Autodesk Fusion 360 part; units mm, degrees
(part 2 of 2)
sketch "Sketch15" plane through (0, 0, 3) normal (0, 0, 1) x (-1, 0, 0)
  line L0 (-1.3462, 92.3209) -> (-1.3462, 60.3952)
  line L1 (-1.3462, 60.3952) -> (-51.7, 11.7691)
  line L2 (-51.7, 11.7691) -> (-51.7, -47.6791)
  line L3 (-51.7, -47.6791) -> (-52.7, -47.6791)
  line L4 (-52.7, -47.6791) -> (-52.7, 12.1936)
  line L5 (-52.7, 12.1936) -> (-2.3462, 60.8196)
  line L6 (-2.3462, 60.8196) -> (-2.3462, 92.3209)
  line L7 (-2.3462, 92.3209) -> (-4.4462, 92.3209)
  line L8 (-4.4462, 92.3209) -> (-4.4462, 61.711)
  line L9 (-4.4462, 61.711) -> (-54.8, 13.085)
  line L10 (-54.8, 13.085) -> (-54.8, -47.6791)
  line L11 (-54.8, -47.6791) -> (-55.8, -47.6791)
  line L12 (-55.8, -47.6791) -> (-55.8, -26.7291)
  line L13 (-55.8, -26.7291) -> (-58.8, -26.7291)
  line L14 (-58.8, -26.7291) -> (-58.8, -18.6291)
  line L15 (-58.8, -18.6291) -> (-55.8, -18.6291)
  line L16 (-55.8, -18.6291) -> (-55.8, 13.5094)
  line L17 (-55.8, 13.5094) -> (-33.2311, 35.304)
  line L18 (-33.2311, 35.304) -> (-35.3151, 37.462)
  line L19 (-35.3151, 37.462) -> (-29.4884, 43.0887)
  line L20 (-29.4884, 43.0887) -> (-27.4044, 40.9307)
  line L21 (-27.4044, 40.9307) -> (-5.4462, 62.1355)
  line L22 (-5.4462, 62.1355) -> (-5.4462, 77.7709)
  line L23 (-5.4462, 77.7709) -> (-8.4462, 77.7709)
  line L24 (-8.4462, 77.7709) -> (-8.4462, 85.8709)
  line L25 (-8.4462, 85.8709) -> (-5.4462, 85.8709)
  line L26 (-5.4462, 85.8709) -> (-5.4462, 92.3209)
  line L27 (-5.4462, 92.3209) -> (-12.45, 92.3209)
  line L28 (-12.45, 92.3209) -> (-12.45, 88.3209)
  line L29 (-12.45, 88.3209) -> (-20.55, 88.3209)
  line L30 (-20.55, 88.3209) -> (-20.55, 92.3209)
  line L31 (-20.55, 92.3209) -> (-71.45, 92.3209)
  line L32 (-71.45, 92.3209) -> (-71.45, 88.3209)
  line L33 (-71.45, 88.3209) -> (-79.55, 88.3209)
  line L34 (-79.55, 88.3209) -> (-79.55, 92.3209)
  line L35 (-79.55, 92.3209) -> (-86.5, 92.3209)
  line L36 (-86.5, 92.3209) -> (-86.5, 85.8709)
  line L37 (-86.5, 85.8709) -> (-82.5, 85.8709)
  line L38 (-82.5, 85.8709) -> (-82.5, 77.7709)
  line L39 (-82.5, 77.7709) -> (-86.5, 77.7709)
  line L40 (-86.5, 77.7709) -> (-86.5, 5.6048)
  line L41 (-86.5, 5.6048) -> (-82.5, 5.6048)
  line L42 (-82.5, 5.6048) -> (-82.5, -2.4952)
  line L43 (-82.5, -2.4952) -> (-86.5, -2.4952)
  line L44 (-86.5, -2.4952) -> (-86.5, -73.6699)
  line L45 (-86.5, -73.6699) -> (-82.5, -73.6699)
  line L46 (-82.5, -73.6699) -> (-82.5, -81.7699)
  line L47 (-82.5, -81.7699) -> (-86.5, -81.7699)
  line L48 (-86.5, -81.7699) -> (-86.5, -88.2199)
  line L49 (-86.5, -88.2199) -> (-79.55, -88.2199)
  line L50 (-79.55, -88.2199) -> (-79.55, -84.2199)
  line L51 (-79.55, -84.2199) -> (-71.45, -84.2199)
  line L52 (-71.45, -84.2199) -> (-71.45, -88.2199)
  line L53 (-71.45, -88.2199) -> (-51.55, -88.2199)
  line L54 (-51.55, -88.2199) -> (-51.55, -84.2199)
  line L55 (-51.55, -84.2199) -> (-43.45, -84.2199)
  line L56 (-43.45, -84.2199) -> (-43.45, -88.2199)
  line L57 (-43.45, -88.2199) -> (-36.5, -88.2199)
  line L58 (-36.5, -88.2199) -> (-36.5, -87.7699)
  line L59 (-36.5, -87.7699) -> (-40.5, -87.7699)
  line L60 (-40.5, -87.7699) -> (-40.5, -79.6699)
  line L61 (-40.5, -79.6699) -> (-36.5, -79.6699)
  line L62 (-36.5, -79.6699) -> (-36.5, -71.6718)
  line L63 (-36.5, -71.6718) -> (-40.5, -71.6718)
  line L64 (-40.5, -71.6718) -> (-40.5, -63.5718)
  line L65 (-40.5, -63.5718) -> (-36.5, -63.5718)
  line L66 (-36.5, -63.5718) -> (-36.5, -63.2199)
  line L67 (-36.5, -63.2199) -> (-36.2957, -62.8659)
  line L68 (-36.2957, -62.8659) -> (-39.7598, -60.8659)
  line L69 (-39.7598, -60.8659) -> (-35.7098, -53.8511)
  line L70 (-35.7098, -53.8511) -> (-32.2457, -55.8511)
  line L71 (-32.2457, -55.8511) -> (-4.298, -7.4443)
  line L72 (-4.298, -7.4443) -> (-7.7621, -5.4443)
  line L73 (-7.7621, -5.4443) -> (-3.7121, 1.5705)
  line L74 (-3.7121, 1.5705) -> (-0.248, -0.4295)
  line L75 (-0.248, -0.4295) -> (0, 0)
  line L76 (0, 0) -> (0.466, 0.1696)
  line L77 (0.466, 0.1696) -> (-0.902, 3.9284)
  line L78 (-0.902, 3.9284) -> (6.7095, 6.6988)
  line L79 (6.7095, 6.6988) -> (8.0776, 2.94)
  line L80 (8.0776, 2.94) -> (80.344, 29.2428)
  line L81 (80.344, 29.2428) -> (78.9759, 33.0016)
  line L82 (78.9759, 33.0016) -> (86.5874, 35.772)
  line L83 (86.5874, 35.772) -> (87.9555, 32.0132)
  line L84 (87.9555, 32.0132) -> (88.801, 32.3209)
  line L85 (88.801, 32.3209) -> (88.801, 36.2709)
  line L86 (88.801, 36.2709) -> (84.801, 36.2709)
  line L87 (84.801, 36.2709) -> (84.801, 44.3709)
  line L88 (84.801, 44.3709) -> (88.801, 44.3709)
  line L89 (88.801, 44.3709) -> (88.801, 83.7709)
  line L90 (88.801, 83.7709) -> (84.801, 83.7709)
  line L91 (84.801, 83.7709) -> (84.801, 91.8709)
  line L92 (84.801, 91.8709) -> (88.801, 91.8709)
  line L93 (88.801, 91.8709) -> (88.801, 92.3209)
  line L94 (88.801, 92.3209) -> (81.851, 92.3209)
  line L95 (81.851, 92.3209) -> (81.851, 88.3209)
  line L96 (81.851, 88.3209) -> (73.751, 88.3209)
  line L97 (73.751, 88.3209) -> (73.751, 92.3209)
  line L98 (73.751, 92.3209) -> (-1.3462, 92.3209)
  line L99 (75, 65) -> (70, 65)
  line L100 (70, 65) -> (70, 40)
  line L101 (70, 40) -> (75, 40)
  line L102 (75, 40) -> (75, 65)
  line L103 (75, 40) -> (35, 40)
  line L104 (35, 40) -> (35, 45)
  line L105 (35, 45) -> (75, 45)
  line L106 (75, 45) -> (75, 40)
  line L107 (65, 50) -> (60, 50)
  line L108 (60, 50) -> (60, 65)
  line L109 (60, 65) -> (65, 65)
  line L110 (65, 65) -> (65, 50)
  line L111 (55, 45) -> (50, 45)
  line L112 (50, 45) -> (50, 55)
  line L113 (50, 55) -> (55, 55)
  line L114 (55, 55) -> (55, 45)
  line L115 (55, 55) -> (35, 55)
  line L116 (35, 55) -> (35, 50)
  line L117 (35, 50) -> (55, 50)
  line L118 (55, 50) -> (55, 55)
  line L119 (35, 50) -> (40, 50)
  line L120 (40, 50) -> (40, 65)
  line L121 (40, 65) -> (35, 65)
  line L122 (35, 65) -> (35, 50)
  line L123 (35, 65) -> (65, 65)
  line L124 (65, 65) -> (65, 60)
  line L125 (65, 60) -> (35, 60)
  line L126 (35, 60) -> (35, 65)
  line L127 (30, 40) -> (25, 40)
  line L128 (25, 40) -> (25, 45)
  line L129 (25, 45) -> (30, 45)
  line L130 (30, 45) -> (30, 40)
  line L131 (30, 50) -> (25, 50)
  line L132 (25, 50) -> (25, 55)
  line L133 (25, 55) -> (30, 55)
  line L134 (30, 55) -> (30, 50)
  line L135 (30, 60) -> (25, 60)
  line L136 (25, 60) -> (25, 65)
  line L137 (25, 65) -> (30, 65)
  line L138 (30, 65) -> (30, 60)
  line L139 (74.99, 67.4454) -> (74.0541, 67.4454)
  line L140 (74.0541, 67.4454) -> (72.8031, 71.0457)
  line L141 (72.8031, 71.0457) -> (72.784, 71.0457)
  line L142 (72.784, 71.0457) -> (71.5425, 67.4454)
  line L143 (71.5425, 67.4454) -> (70.597, 67.4454)
  line L144 (70.597, 67.4454) -> (70.597, 74.245)
  line L145 (70.597, 74.245) -> (71.5711, 74.245)
  line L146 (71.5711, 74.245) -> (71.5711, 70.1098)
  line L147 (71.5711, 70.1098) -> (71.5902, 70.1098)
  line L148 (71.5902, 70.1098) -> (72.5548, 73.0321)
  line L149 (72.5548, 73.0321) -> (73.0418, 73.0321)
  line L150 (73.0418, 73.0321) -> (73.9968, 70.1098)
  line L151 (73.9968, 70.1098) -> (74.0159, 70.1098)
  line L152 (74.0159, 70.1098) -> (74.0159, 74.245)
  line L153 (74.0159, 74.245) -> (74.99, 74.245)
  line L154 (74.99, 74.245) -> (74.99, 67.4454)
  line L155 (69.6515, 67.4454) -> (68.6775, 67.4454)
  line L156 (68.6775, 67.4454) -> (68.6775, 74.245)
  line L157 (68.6775, 74.245) -> (69.6515, 74.245)
  line L158 (69.6515, 74.245) -> (69.6515, 67.4454)
  line L159 (67.732, 67.4454) -> (66.7579, 67.4454)
  line L160 (66.7579, 67.4454) -> (66.7579, 73.2709)
  line L161 (66.7579, 73.2709) -> (64.8288, 73.2709)
  line L162 (64.8288, 73.2709) -> (64.8288, 74.245)
  line L163 (64.8288, 74.245) -> (67.732, 74.245)
  line L164 (67.732, 74.245) -> (67.732, 67.4454)
  line L165 (64.1985, 67.4454) -> (61.2953, 67.4454)
  line L166 (61.2953, 67.4454) -> (61.2953, 68.3622)
  line L167 (61.2953, 68.3622) -> (63.2244, 68.3622)
  line L168 (63.2244, 68.3622) -> (63.2244, 70.3581)
  line L169 (63.2244, 70.3581) -> (61.5436, 70.3581)
  line L170 (61.5436, 70.3581) -> (61.5436, 71.2749)
  line L171 (61.5436, 71.2749) -> (63.2244, 71.2749)
  line L172 (63.2244, 71.2749) -> (63.2244, 73.2709)
  line L173 (63.2244, 73.2709) -> (61.2953, 73.2709)
  line L174 (61.2953, 73.2709) -> (61.2953, 74.245)
  line L175 (61.2953, 74.245) -> (64.1985, 74.245)
  line L176 (64.1985, 74.245) -> (64.1985, 67.4454)
  line L177 (57.5135, 69.4031) -> (58.4876, 69.4031)
  line L178 (58.4876, 69.4031) -> (58.4876, 69.1835)
  spline S0 degree 3 poles (58.4876, 69.1835) (58.4932, 69.0777) (58.5041, 68.8742) (58.6026, 68.6961) (58.65, 68.6105) knots 0 0 0 0 0.031302 0.06025 0.06025 0.06025 0.06025
  spline S1 degree 3 poles (58.65, 68.6105) (58.7141, 68.5382) (58.8526, 68.382) (59.0625, 68.3691) (59.1752, 68.3622) knots 0 0 0 0 0.027897 0.060252 0.060252 0.060252 0.060252
  spline S2 degree 3 poles (59.1752, 68.3622) (59.2375, 68.3644) (59.354, 68.3685) (59.4601, 68.4163) (59.5095, 68.4386) knots 0 0 0 0 0.018483 0.034579 0.034579 0.034579 0.034579
  spline S3 degree 3 poles (59.5095, 68.4386) (59.5488, 68.466) (59.6276, 68.5209) (59.6825, 68.5997) (59.71, 68.6391) knots 0 0 0 0 0.014281 0.028562 0.028562 0.028562 0.028562
  spline S4 degree 3 poles (59.71, 68.6391) (59.7309, 68.6807) (59.7752, 68.7686) (59.795, 68.8651) (59.8055, 68.9161) knots 0 0 0 0 0.013891 0.029409 0.029409 0.029409 0.029409
  spline S5 degree 3 poles (59.8055, 68.9161) (59.8139, 68.9685) (59.831, 69.076) (59.8331, 69.1849) (59.8342, 69.2408) knots 0 0 0 0 0.015903 0.032631 0.032631 0.032631 0.032631
  spline S6 degree 3 poles (59.8342, 69.2408) (59.8339, 69.3029) (59.8334, 69.4175) (59.8274, 69.5321) (59.8246, 69.5846) knots 0 0 0 0 0.018624 0.034398 0.034398 0.034398 0.034398
  spline S7 degree 3 poles (59.8246, 69.5846) (59.817, 69.6274) (59.8021, 69.7104) (59.7658, 69.7865) (59.7482, 69.8233) knots 0 0 0 0 0.012974 0.025169 0.025169 0.025169 0.025169
  spline S8 degree 3 poles (59.7482, 69.8233) (59.7265, 69.8548) (59.6812, 69.9204) (59.6185, 69.9696) (59.5858, 69.9952) knots 0 0 0 0 0.011413 0.023766 0.023766 0.023766 0.023766
  spline S9 degree 3 poles (59.5858, 69.9952) (59.5418, 70.0217) (59.444, 70.0806) (59.3383, 70.1241) (59.2803, 70.148) knots 0 0 0 0 0.015399 0.03421 0.03421 0.03421 0.03421
  line L179 (59.2803, 70.148) -> (58.5353, 70.4441)
  spline S10 degree 3 poles (58.5353, 70.4441) (58.435, 70.4852) (58.2475, 70.562) (58.0855, 70.6836) (58.0101, 70.7401) knots 0 0 0 0 0.032366 0.060512 0.060512 0.060512 0.060512
  spline S11 degree 3 poles (58.0101, 70.7401) (57.9473, 70.7968) (57.8226, 70.9095) (57.7437, 71.0579) (57.7045, 71.1317) knots 0 0 0 0 0.025155 0.050009 0.050009 0.050009 0.050009
  spline S12 degree 3 poles (57.7045, 71.1317) (57.6692, 71.2102) (57.5951, 71.3752) (57.5666, 71.5538) (57.5517, 71.6474) knots 0 0 0 0 0.025714 0.053996 0.053996 0.053996 0.053996
  spline S13 degree 3 poles (57.5517, 71.6474) (57.5406, 71.7499) (57.5168, 71.9689) (57.5146, 72.1892) (57.5135, 72.3063) knots 0 0 0 0 0.030932 0.066041 0.066041 0.066041 0.066041
  spline S14 degree 3 poles (57.5135, 72.3063) (57.5166, 72.4452) (57.5227, 72.7151) (57.5744, 72.98) (57.5994, 73.1085) knots 0 0 0 0 0.041598 0.080809 0.080809 0.080809 0.080809
  spline S15 degree 3 poles (57.5994, 73.1085) (57.6319, 73.2242) (57.695, 73.4491) (57.8235, 73.6441) (57.8859, 73.7388) knots 0 0 0 0 0.035787 0.069609 0.069609 0.069609 0.069609
  spline S16 degree 3 poles (57.8859, 73.7388) (57.9567, 73.8211) (58.1024, 73.9906) (58.3, 74.0955) (58.4017, 74.1495) knots 0 0 0 0 0.032249 0.06644 0.06644 0.06644 0.06644
  spline S17 degree 3 poles (58.4017, 74.1495) (58.5206, 74.194) (58.7758, 74.2895) (59.0486, 74.2978) (59.1943, 74.3023) knots 0 0 0 0 0.037829 0.081211 0.081211 0.081211 0.081211
  spline S18 degree 3 poles (59.1943, 74.3023) (59.3092, 74.2975) (59.5349, 74.2881) (59.7484, 74.2143) (59.8532, 74.1781) knots 0 0 0 0 0.034282 0.067373 0.067373 0.067373 0.067373
  spline S19 degree 3 poles (59.8532, 74.1781) (59.9507, 74.1339) (60.1417, 74.0473) (60.3007, 73.9107) (60.3785, 73.8439) knots 0 0 0 0 0.031927 0.06254 0.06254 0.06254 0.06254
  spline S20 degree 3 poles (60.3785, 73.8439) (60.4484, 73.7669) (60.5898, 73.6112) (60.6841, 73.4232) (60.7318, 73.3282) knots 0 0 0 0 0.031027 0.062774 0.062774 0.062774 0.062774
  spline S21 degree 3 poles (60.7318, 73.3282) (60.7681, 73.2265) (60.8418, 73.0196) (60.8512, 72.8) (60.856, 72.6883) knots 0 0 0 0 0.032175 0.065507 0.065507 0.065507 0.065507
  line L180 (60.856, 72.6883) -> (60.856, 72.3254)
  line L181 (60.856, 72.3254) -> (59.8819, 72.3254)
  line L182 (59.8819, 72.3254) -> (59.8819, 72.631)
  spline S22 degree 3 poles (59.8819, 72.631) (59.8755, 72.7182) (59.8628, 72.8925) (59.7737, 73.0429) (59.7291, 73.1181) knots 0 0 0 0 0.02583 0.051669 0.051669 0.051669 0.051669
  spline S23 degree 3 poles (59.7291, 73.1181) (59.6611, 73.1792) (59.5103, 73.3147) (59.3063, 73.3234) (59.1943, 73.3282) knots 0 0 0 0 0.026646 0.059067 0.059067 0.059067 0.059067
  spline S24 degree 3 poles (59.1943, 73.3282) (59.1202, 73.3271) (58.989, 73.3253) (58.8659, 73.2807) (58.8123, 73.2613) knots 0 0 0 0 0.022028 0.03902 0.03902 0.03902 0.03902
  spline S25 degree 3 poles (58.8123, 73.2613) (58.7682, 73.2347) (58.6832, 73.1834) (58.6285, 73.1006) (58.6022, 73.0608) knots 0 0 0 0 0.015237 0.029372 0.029372 0.029372 0.029372
  spline S26 degree 3 poles (58.6022, 73.0608) (58.579, 73.0122) (58.5297, 72.9092) (58.5147, 72.7959) (58.5067, 72.7361) knots 0 0 0 0 0.016051 0.034032 0.034032 0.034032 0.034032
  spline S27 degree 3 poles (58.5067, 72.7361) (58.5011, 72.6693) (58.4895, 72.5294) (58.4882, 72.3891) (58.4876, 72.3159) knots 0 0 0 0 0.020106 0.042076 0.042076 0.042076 0.042076
  spline S28 degree 3 poles (58.4876, 72.3159) (58.488, 72.2346) (58.4887, 72.088) (58.5011, 71.9418) (58.5067, 71.8766) knots 0 0 0 0 0.024357 0.043987 0.043987 0.043987 0.043987
  spline S29 degree 3 poles (58.5067, 71.8766) (58.514, 71.8239) (58.5274, 71.7267) (58.5722, 71.6395) (58.5926, 71.5996) knots 0 0 0 0 0.015826 0.029183 0.029183 0.029183 0.029183
  spline S30 degree 3 poles (58.5926, 71.5996) (58.6146, 71.5659) (58.6598, 71.4966) (58.729, 71.4511) (58.7645, 71.4277) knots 0 0 0 0 0.011937 0.024544 0.024544 0.024544 0.024544
  spline S31 degree 3 poles (58.7645, 71.4277) (58.8055, 71.4039) (58.898, 71.3501) (58.9963, 71.308) (59.0511, 71.2845) knots 0 0 0 0 0.014215 0.032058 0.032058 0.032058 0.032058
  line L183 (59.0511, 71.2845) -> (59.7482, 70.998)
  spline S32 degree 3 poles (59.7482, 70.998) (59.9365, 70.9135) (60.2794, 70.7595) (60.4991, 70.4566) (60.5981, 70.3199) knots 0 0 0 0 0.060619 0.110418 0.110418 0.110418 0.110418
  spline S33 degree 3 poles (60.5981, 70.3199) (60.6593, 70.1609) (60.7916, 69.8172) (60.8024, 69.4485) (60.8082, 69.2503) knots 0 0 0 0 0.050736 0.109703 0.109703 0.109703 0.109703
  spline S34 degree 3 poles (60.8082, 69.2503) (60.8041, 69.1255) (60.7961, 68.8796) (60.7338, 68.6417) (60.7032, 68.5245) knots 0 0 0 0 0.037337 0.07354 0.07354 0.07354 0.07354
  spline S35 degree 3 poles (60.7032, 68.5245) (60.6653, 68.4153) (60.5917, 68.2032) (60.461, 68.0208) (60.3976, 67.9324) knots 0 0 0 0 0.034493 0.066942 0.066942 0.066942 0.066942
  spline S36 degree 3 poles (60.3976, 67.9324) (60.3224, 67.8537) (60.1694, 67.6936) (59.9724, 67.5923) (59.8723, 67.5409) knots 0 0 0 0 0.03243 0.065924 0.065924 0.065924 0.065924
  spline S37 degree 3 poles (59.8723, 67.5409) (59.7599, 67.4963) (59.5239, 67.4028) (59.2699, 67.3932) (59.137, 67.3881) knots 0 0 0 0 0.036013 0.075592 0.075592 0.075592 0.075592
  spline S38 degree 3 poles (59.137, 67.3881) (59.0203, 67.393) (58.7934, 67.4025) (58.5812, 67.4828) (58.478, 67.5218) knots 0 0 0 0 0.03478 0.067624 0.067624 0.067624 0.067624
  spline S39 degree 3 poles (58.478, 67.5218) (58.381, 67.569) (58.1916, 67.6613) (58.0375, 67.805) (57.9623, 67.8751) knots 0 0 0 0 0.032164 0.062825 0.062825 0.062825 0.062825
  spline S40 degree 3 poles (57.9623, 67.8751) (57.8937, 67.9503) (57.7576, 68.0993) (57.671, 68.2815) (57.6281, 68.3717) knots 0 0 0 0 0.030355 0.060157 0.060157 0.060157 0.060157
  spline S41 degree 3 poles (57.6281, 68.3717) (57.5947, 68.4615) (57.5281, 68.6402) (57.5183, 68.8307) (57.5135, 68.9256) knots 0 0 0 0 0.028542 0.05686 0.05686 0.05686 0.05686
  line L184 (57.5135, 68.9256) -> (57.5135, 69.4031)
  line L185 (56.1479, 68.3622) -> (57.2748, 68.3622)
  line L186 (57.2748, 68.3622) -> (57.2748, 67.4454)
  line L187 (57.2748, 67.4454) -> (54.0469, 67.4454)
  line L188 (54.0469, 67.4454) -> (54.0469, 68.3622)
  line L189 (54.0469, 68.3622) -> (55.1738, 68.3622)
  line L190 (55.1738, 68.3622) -> (55.1738, 74.245)
  line L191 (55.1738, 74.245) -> (56.1479, 74.245)
  line L192 (56.1479, 74.245) -> (56.1479, 68.3622)
  spline S42 degree 3 poles (53.6744, 69.0498) (53.6696, 68.9194) (53.6603, 68.6697) (53.5729, 68.4358) (53.5311, 68.324) knots 0 0 0 0 0.038843 0.074407 0.074407 0.074407 0.074407
  spline S43 degree 3 poles (53.5311, 68.324) (53.4812, 68.2249) (53.3844, 68.0331) (53.2322, 67.8815) (53.1587, 67.8083) knots 0 0 0 0 0.033049 0.06398 0.06398 0.06398 0.06398
  spline S44 degree 3 poles (53.1587, 67.8083) (53.0776, 67.7428) (52.9172, 67.6133) (52.7274, 67.5329) (52.6334, 67.4931) knots 0 0 0 0 0.031087 0.061522 0.061522 0.061522 0.061522
  spline S45 degree 3 poles (52.6334, 67.4931) (52.5355, 67.4625) (52.3426, 67.4021) (52.1408, 67.3927) (52.0413, 67.3881) knots 0 0 0 0 0.030635 0.060357 0.060357 0.060357 0.060357
  spline S46 degree 3 poles (52.0413, 67.3881) (51.9427, 67.3926) (51.7439, 67.4017) (51.5543, 67.4625) (51.4588, 67.4931) knots 0 0 0 0 0.029483 0.059427 0.059427 0.059427 0.059427
  spline S47 degree 3 poles (51.4588, 67.4931) (51.363, 67.5324) (51.1719, 67.6108) (51.0129, 67.7426) (50.9335, 67.8083) knots 0 0 0 0 0.030866 0.06157 0.06157 0.06157 0.06157
  spline S48 degree 3 poles (50.9335, 67.8083) (50.8573, 67.8813) (50.7007, 68.0313) (50.6021, 68.2247) (50.5515, 68.324) knots 0 0 0 0 0.031417 0.064585 0.064585 0.064585 0.064585
  spline S49 degree 3 poles (50.5515, 68.324) (50.5098, 68.4358) (50.4224, 68.6697) (50.4131, 68.9194) (50.4083, 69.0498) knots 0 0 0 0 0.035564 0.074407 0.074407 0.074407 0.074407
  line L193 (50.4083, 69.0498) -> (50.4083, 72.6406)
  spline S50 degree 3 poles (50.4083, 72.6406) (50.413, 72.7733) (50.4219, 73.0262) (50.5098, 73.2633) (50.5515, 73.3759) knots 0 0 0 0 0.039556 0.075348 0.075348 0.075348 0.075348
  spline S51 degree 3 poles (50.5515, 73.3759) (50.6027, 73.4733) (50.7033, 73.665) (50.8576, 73.8169) (50.9335, 73.8916) knots 0 0 0 0 0.032757 0.064524 0.064524 0.064524 0.064524
  spline S52 degree 3 poles (50.9335, 73.8916) (51.0131, 73.9546) (51.1735, 74.0817) (51.3632, 74.1585) (51.4588, 74.1972) knots 0 0 0 0 0.03028 0.061045 0.061045 0.061045 0.061045
  spline S53 degree 3 poles (51.4588, 74.1972) (51.5543, 74.2279) (51.7439, 74.2887) (51.9427, 74.2978) (52.0413, 74.3023) knots 0 0 0 0 0.029944 0.059427 0.059427 0.059427 0.059427
  spline S54 degree 3 poles (52.0413, 74.3023) (52.1408, 74.2976) (52.3426, 74.2882) (52.5355, 74.2279) (52.6334, 74.1972) knots 0 0 0 0 0.029721 0.060357 0.060357 0.060357 0.060357
  spline S55 degree 3 poles (52.6334, 74.1972) (52.7272, 74.158) (52.9157, 74.0793) (53.0774, 73.9544) (53.1587, 73.8916) knots 0 0 0 0 0.030333 0.061001 0.061001 0.061001 0.061001
  spline S56 degree 3 poles (53.1587, 73.8916) (53.232, 73.8166) (53.3818, 73.6633) (53.4807, 73.473) (53.5311, 73.3759) knots 0 0 0 0 0.031287 0.063923 0.063923 0.063923 0.063923
  spline S57 degree 3 poles (53.5311, 73.3759) (53.5729, 73.2633) (53.6608, 73.0262) (53.6697, 72.7733) (53.6744, 72.6406) knots 0 0 0 0 0.035792 0.075348 0.075348 0.075348 0.075348
  line L194 (53.6744, 72.6406) -> (53.6744, 69.0498)
  spline S58 degree 3 poles (52.7003, 72.6406) (52.6956, 72.7476) (52.6871, 72.9439) (52.5649, 73.0964) (52.5093, 73.1658) knots 0 0 0 0 0.031167 0.05719 0.05719 0.05719 0.05719
  spline S59 degree 3 poles (52.5093, 73.1658) (52.4392, 73.2132) (52.2977, 73.3088) (52.1274, 73.3217) (52.0413, 73.3282) knots 0 0 0 0 0.024906 0.050301 0.050301 0.050301 0.050301
  spline S60 degree 3 poles (52.0413, 73.3282) (51.956, 73.3219) (51.7882, 73.3096) (51.6506, 73.2132) (51.5829, 73.1658) knots 0 0 0 0 0.025159 0.049443 0.049443 0.049443 0.049443
  spline S61 degree 3 poles (51.5829, 73.1658) (51.5246, 73.0967) (51.3972, 72.9461) (51.3876, 72.7479) (51.3824, 72.6406) knots 0 0 0 0 0.026425 0.057629 0.057629 0.057629 0.057629
  line L195 (51.3824, 72.6406) -> (51.3824, 69.0498)
  spline S62 degree 3 poles (51.3824, 69.0498) (51.3873, 68.943) (51.3963, 68.7472) (51.5246, 68.6007) (51.5829, 68.5341) knots 0 0 0 0 0.030969 0.056808 0.056808 0.056808 0.056808
  spline S63 degree 3 poles (51.5829, 68.5341) (51.6503, 68.4839) (51.7864, 68.3826) (51.9558, 68.369) (52.0413, 68.3622) knots 0 0 0 0 0.02465 0.049849 0.049849 0.049849 0.049849
  spline S64 degree 3 poles (52.0413, 68.3622) (52.1276, 68.3692) (52.2995, 68.3833) (52.4395, 68.4839) (52.5093, 68.5341) knots 0 0 0 0 0.025434 0.050698 0.050698 0.050698 0.050698
  spline S65 degree 3 poles (52.5093, 68.5341) (52.5649, 68.601) (52.688, 68.7494) (52.696, 68.9433) (52.7003, 69.0498) knots 0 0 0 0 0.025429 0.05636 0.05636 0.05636 0.05636
  line L196 (52.7003, 69.0498) -> (52.7003, 72.6406)
  line L197 (48.5747, 70.4823) -> (48.0208, 70.4823)
  spline S66 degree 3 poles (48.0208, 70.4823) (47.9429, 70.481) (47.8025, 70.4786) (47.6694, 70.4349) (47.6102, 70.4154) knots 0 0 0 0 0.023219 0.041814 0.041814 0.041814 0.041814
  spline S67 degree 3 poles (47.6102, 70.4154) (47.5628, 70.3882) (47.4706, 70.3353) (47.4103, 70.2478) (47.3809, 70.2053) knots 0 0 0 0 0.016158 0.031445 0.031445 0.031445 0.031445
  spline S68 degree 3 poles (47.3809, 70.2053) (47.3545, 70.1569) (47.2987, 70.055) (47.2775, 69.9407) (47.2663, 69.8806) knots 0 0 0 0 0.016444 0.034627 0.034627 0.034627 0.034627
  spline S69 degree 3 poles (47.2663, 69.8806) (47.258, 69.8091) (47.2402, 69.6568) (47.2386, 69.5035) (47.2377, 69.4222) knots 0 0 0 0 0.021595 0.045958 0.045958 0.045958 0.045958
  spline S70 degree 3 poles (47.2377, 69.4222) (47.2385, 69.3417) (47.24, 69.1916) (47.258, 69.0425) (47.2663, 68.9734) knots 0 0 0 0 0.024124 0.045006 0.045006 0.045006 0.045006
  spline S71 degree 3 poles (47.2663, 68.9734) (47.2777, 68.9107) (47.2993, 68.7918) (47.3612, 68.6881) (47.3905, 68.6391) knots 0 0 0 0 0.018935 0.035915 0.035915 0.035915 0.035915
  spline S72 degree 3 poles (47.3905, 68.6391) (47.4227, 68.5944) (47.4879, 68.5038) (47.5881, 68.4542) (47.6388, 68.429) knots 0 0 0 0 0.016263 0.032969 0.032969 0.032969 0.032969
  spline S73 degree 3 poles (47.6388, 68.429) (47.7012, 68.4096) (47.8409, 68.3661) (47.9875, 68.3636) (48.0685, 68.3622) knots 0 0 0 0 0.019516 0.043688 0.043688 0.043688 0.043688
  line L198 (48.0685, 68.3622) -> (48.5747, 68.3622)
  line L199 (48.5747, 68.3622) -> (48.5747, 70.4823)
  line L200 (49.5488, 67.4454) -> (47.9826, 67.4454)
  spline S74 degree 3 poles (47.9826, 67.4454) (47.4817, 67.5467) (46.4165, 67.7621) (46.3166, 68.8598) (46.2636, 69.4413) knots 0 0 0 0 0.138244 0.293987 0.293987 0.293987 0.293987
  spline S75 degree 3 poles (46.2636, 69.4413) (46.2695, 69.6271) (46.2806, 69.9779) (46.3989, 70.3079) (46.4546, 70.4632) knots 0 0 0 0 0.055358 0.104524 0.104524 0.104524 0.104524
  spline S76 degree 3 poles (46.4546, 70.4632) (46.5301, 70.5981) (46.6876, 70.8798) (46.9614, 71.0517) (47.104, 71.1412) knots 0 0 0 0 0.045624 0.095236 0.095236 0.095236 0.095236
  line L201 (47.104, 71.1412) -> (46.0535, 74.245)
  line L202 (46.0535, 74.245) -> (47.0849, 74.245)
  line L203 (47.0849, 74.245) -> (47.9921, 71.3418)
  line L204 (47.9921, 71.3418) -> (48.5747, 71.3418)
  line L205 (48.5747, 71.3418) -> (48.5747, 74.245)
  line L206 (48.5747, 74.245) -> (49.5488, 74.245)
  line L207 (49.5488, 74.245) -> (49.5488, 67.4454)
  line L208 (45.4805, 67.4454) -> (44.5446, 67.4454)
  line L209 (44.5446, 67.4454) -> (43.2936, 71.0457)
  line L210 (43.2936, 71.0457) -> (43.2745, 71.0457)
  line L211 (43.2745, 71.0457) -> (42.033, 67.4454)
  line L212 (42.033, 67.4454) -> (41.0875, 67.4454)
  line L213 (41.0875, 67.4454) -> (41.0875, 74.245)
  line L214 (41.0875, 74.245) -> (42.0616, 74.245)
  line L215 (42.0616, 74.245) -> (42.0616, 70.1098)
  line L216 (42.0616, 70.1098) -> (42.0807, 70.1098)
  line L217 (42.0807, 70.1098) -> (43.0453, 73.0321)
  line L218 (43.0453, 73.0321) -> (43.5323, 73.0321)
  line L219 (43.5323, 73.0321) -> (44.4873, 70.1098)
  line L220 (44.4873, 70.1098) -> (44.5064, 70.1098)
  line L221 (44.5064, 70.1098) -> (44.5064, 74.245)
  line L222 (44.5064, 74.245) -> (45.4805, 74.245)
  line L223 (45.4805, 74.245) -> (45.4805, 67.4454)
  line L224 (38.5281, 73.3282) -> (36.7709, 70.0143)
  spline S77 degree 3 poles (36.7709, 70.0143) (36.7317, 69.9386) (36.661, 69.8021) (36.6313, 69.6516) (36.6181, 69.5846) knots 0 0 0 0 0.02543 0.045813 0.045813 0.045813 0.045813
  spline S78 degree 3 poles (36.6181, 69.5846) (36.6125, 69.5138) (36.6003, 69.358) (36.5995, 69.2018) (36.599, 69.1166) knots 0 0 0 0 0.021297 0.046848 0.046848 0.046848 0.046848
  spline S79 degree 3 poles (36.599, 69.1166) (36.5994, 69.0744) (36.6003, 68.9884) (36.6058, 68.9025) (36.6085, 68.8588) knots 0 0 0 0 0.012656 0.025807 0.025807 0.025807 0.025807
  spline S80 degree 3 poles (36.6085, 68.8588) (36.6128, 68.8137) (36.621, 68.7284) (36.6515, 68.6483) (36.6659, 68.6105) knots 0 0 0 0 0.013506 0.025586 0.025586 0.025586 0.025586
  spline S81 degree 3 poles (36.6659, 68.6105) (36.6811, 68.5769) (36.7121, 68.5091) (36.7702, 68.4623) (36.7995, 68.4386) knots 0 0 0 0 0.010899 0.022046 0.022046 0.022046 0.022046
  spline S82 degree 3 poles (36.7995, 68.4386) (36.8376, 68.4164) (36.9228, 68.3667) (37.0218, 68.3638) (37.0765, 68.3622) knots 0 0 0 0 0.013027 0.029137 0.029137 0.029137 0.029137
  spline S83 degree 3 poles (37.0765, 68.3622) (37.1448, 68.3662) (37.2749, 68.3739) (37.38, 68.4501) (37.4298, 68.4863) knots 0 0 0 0 0.020058 0.038156 0.038156 0.038156 0.038156
  spline S84 degree 3 poles (37.4298, 68.4863) (37.466, 68.5354) (37.545, 68.6428) (37.5508, 68.7766) (37.554, 68.8492) knots 0 0 0 0 0.017893 0.039132 0.039132 0.039132 0.039132
  line L225 (37.554, 68.8492) -> (37.554, 69.4031)
  line L226 (37.554, 69.4031) -> (38.5281, 69.4031)
  line L227 (38.5281, 69.4031) -> (38.5281, 68.8683)
  spline S85 degree 3 poles (38.5281, 68.8683) (38.5236, 68.7686) (38.5146, 68.5717) (38.4469, 68.3867) (38.4135, 68.2953) knots 0 0 0 0 0.029743 0.058741 0.058741 0.058741 0.058741
  spline S86 degree 3 poles (38.4135, 68.2953) (38.3725, 68.2094) (38.2916, 68.0397) (38.1686, 67.8976) (38.1079, 67.8274) knots 0 0 0 0 0.028411 0.056116 0.056116 0.056116 0.056116
  spline S87 degree 3 poles (38.1079, 67.8274) (38.038, 67.764) (37.8972, 67.6364) (37.7261, 67.5538) (37.64, 67.5122) knots 0 0 0 0 0.028154 0.056679 0.056679 0.056679 0.056679
  spline S88 degree 3 poles (37.64, 67.5122) (37.5488, 67.476) (37.3647, 67.4029) (37.1668, 67.3931) (37.0669, 67.3881) knots 0 0 0 0 0.029219 0.058986 0.058986 0.058986 0.058986
  spline S89 degree 3 poles (37.0669, 67.3881) (36.9474, 67.3925) (36.722, 67.4008) (36.5149, 67.4896) (36.4176, 67.5313) knots 0 0 0 0 0.035516 0.06701 0.06701 0.06701 0.06701
  spline S90 degree 3 poles (36.4176, 67.5313) (36.33, 67.5798) (36.1568, 67.6756) (36.0309, 67.8283) (35.9687, 67.9038) knots 0 0 0 0 0.029737 0.058792 0.058792 0.058792 0.058792
  spline S91 degree 3 poles (35.9687, 67.9038) (35.9124, 67.9868) (35.7985, 68.1549) (35.7403, 68.3496) (35.7109, 68.4481) knots 0 0 0 0 0.02989 0.060549 0.060549 0.060549 0.060549
  spline S92 degree 3 poles (35.7109, 68.4481) (35.6858, 68.5527) (35.6346, 68.7662) (35.6282, 68.9856) (35.6249, 69.0975) knots 0 0 0 0 0.032168 0.065662 0.065662 0.065662 0.065662
  spline S93 degree 3 poles (35.6249, 69.0975) (35.6251, 69.1739) (35.6256, 69.3141) (35.6317, 69.4541) (35.6344, 69.5177) knots 0 0 0 0 0.022921 0.042035 0.042035 0.042035 0.042035
  spline S94 degree 3 poles (35.6344, 69.5177) (35.6384, 69.5712) (35.6461, 69.6768) (35.6639, 69.7812) (35.6726, 69.8329) knots 0 0 0 0 0.01606 0.031762 0.031762 0.031762 0.031762
  spline S95 degree 3 poles (35.6726, 69.8329) (35.684, 69.8842) (35.7071, 69.9888) (35.7475, 70.088) (35.7682, 70.1385) knots 0 0 0 0 0.01575 0.032069 0.032069 0.032069 0.032069
  spline S96 degree 3 poles (35.7682, 70.1385) (35.794, 70.1952) (35.8513, 70.3209) (35.9148, 70.4436) (35.9496, 70.5109) knots 0 0 0 0 0.018693 0.041435 0.041435 0.041435 0.041435
  line L228 (35.9496, 70.5109) -> (37.3821, 73.2709)
  line L229 (37.3821, 73.2709) -> (35.6249, 73.2709)
  line L230 (35.6249, 73.2709) -> (35.6249, 74.245)
  line L231 (35.6249, 74.245) -> (38.5281, 74.245)
  line L232 (38.5281, 74.245) -> (38.5281, 73.3282)
  spline S97 degree 3 poles (34.9755, 68.8492) (34.9716, 68.7399) (34.9641, 68.5303) (34.8943, 68.3326) (34.8609, 68.238) knots 0 0 0 0 0.032596 0.062508 0.062508 0.062508 0.062508
  spline S98 degree 3 poles (34.8609, 68.238) (34.8169, 68.1526) (34.7302, 67.9845) (34.6002, 67.8472) (34.5362, 67.7796) knots 0 0 0 0 0.028666 0.056427 0.056427 0.056427 0.056427
  spline S99 degree 3 poles (34.5362, 67.7796) (34.467, 67.72) (34.329, 67.6009) (34.1614, 67.529) (34.0778, 67.4931) knots 0 0 0 0 0.027222 0.054343 0.054343 0.054343 0.054343
  spline S100 degree 3 poles (34.0778, 67.4931) (33.9879, 67.4625) (33.8082, 67.4013) (33.6186, 67.3925) (33.5239, 67.3881) knots 0 0 0 0 0.028335 0.056629 0.056629 0.056629 0.056629
  spline S101 degree 3 poles (33.5239, 67.3881) (33.4299, 67.3923) (33.2433, 67.4008) (33.067, 67.4625) (32.9795, 67.4931) knots 0 0 0 0 0.028057 0.055705 0.055705 0.055705 0.055705
  spline S102 degree 3 poles (32.9795, 67.4931) (32.8934, 67.5287) (32.7223, 67.5995) (32.5815, 67.7198) (32.5116, 67.7796) knots 0 0 0 0 0.027766 0.055176 0.055176 0.055176 0.055176
  spline S103 degree 3 poles (32.5116, 67.7796) (32.4481, 67.847) (32.3195, 67.9836) (32.2378, 68.1525) (32.1964, 68.238) knots 0 0 0 0 0.027605 0.05592 0.05592 0.05592 0.05592
  spline S104 degree 3 poles (32.1964, 68.238) (32.1603, 68.3325) (32.0849, 68.5291) (32.0766, 68.7397) (32.0723, 68.8492) knots 0 0 0 0 0.030125 0.062743 0.062743 0.062743 0.062743
  line L233 (32.0723, 68.8492) -> (32.0723, 72.8411)
  spline S105 degree 3 poles (32.0723, 72.8411) (32.0766, 72.9506) (32.0849, 73.1612) (32.1603, 73.3579) (32.1964, 73.4523) knots 0 0 0 0 0.032618 0.062743 0.062743 0.062743 0.062743
  spline S106 degree 3 poles (32.1964, 73.4523) (32.2378, 73.5379) (32.3195, 73.7068) (32.4481, 73.8433) (32.5116, 73.9107) knots 0 0 0 0 0.028315 0.05592 0.05592 0.05592 0.05592
  spline S107 degree 3 poles (32.5116, 73.9107) (32.5816, 73.971) (32.7231, 74.0926) (32.8935, 74.1685) (32.9795, 74.2068) knots 0 0 0 0 0.027557 0.055638 0.055638 0.055638 0.055638
  spline S108 degree 3 poles (32.9795, 74.2068) (33.0672, 74.2346) (33.2443, 74.2909) (33.4301, 74.2985) (33.5239, 74.3023) knots 0 0 0 0 0.027452 0.055488 0.055488 0.055488 0.055488
  spline S109 degree 3 poles (33.5239, 74.3023) (33.6185, 74.2983) (33.8073, 74.2905) (33.9878, 74.2346) (34.0778, 74.2068) knots 0 0 0 0 0.028273 0.056418 0.056418 0.056418 0.056418
  spline S110 degree 3 poles (34.0778, 74.2068) (34.1613, 74.1682) (34.3281, 74.0912) (34.4669, 73.9708) (34.5362, 73.9107) knots 0 0 0 0 0.027444 0.054813 0.054813 0.054813 0.054813
  spline S111 degree 3 poles (34.5362, 73.9107) (34.6002, 73.8432) (34.7302, 73.7059) (34.8169, 73.5377) (34.8609, 73.4523) knots 0 0 0 0 0.027761 0.056427 0.056427 0.056427 0.056427
  spline S112 degree 3 poles (34.8609, 73.4523) (34.8943, 73.3577) (34.9641, 73.1601) (34.9716, 72.9504) (34.9755, 72.8411) knots 0 0 0 0 0.029912 0.062508 0.062508 0.062508 0.062508
  line L234 (34.9755, 72.8411) -> (34.9755, 68.8492)
  spline S113 degree 3 poles (34.0014, 72.8411) (33.9963, 72.9079) (33.9862, 73.0389) (33.9067, 73.1433) (33.8677, 73.1945) knots 0 0 0 0 0.019626 0.038505 0.038505 0.038505 0.038505
  spline S114 degree 3 poles (33.8677, 73.1945) (33.819, 73.2335) (33.7185, 73.3138) (33.59, 73.3233) (33.5239, 73.3282) knots 0 0 0 0 0.018276 0.037667 0.037667 0.037667 0.037667
  spline S115 degree 3 poles (33.5239, 73.3282) (33.4578, 73.3233) (33.3293, 73.3138) (33.2288, 73.2335) (33.1801, 73.1945) knots 0 0 0 0 0.01939 0.037667 0.037667 0.037667 0.037667
  spline S116 degree 3 poles (33.1801, 73.1945) (33.1411, 73.1433) (33.0616, 73.0389) (33.0515, 72.9079) (33.0464, 72.8411) knots 0 0 0 0 0.018879 0.038505 0.038505 0.038505 0.038505
  line L235 (33.0464, 72.8411) -> (33.0464, 68.8492)
  spline S117 degree 3 poles (33.0464, 68.8492) (33.0513, 68.7831) (33.0608, 68.6546) (33.1411, 68.5542) (33.1801, 68.5054) knots 0 0 0 0 0.01939 0.037667 0.037667 0.037667 0.037667
  spline S118 degree 3 poles (33.1801, 68.5054) (33.2285, 68.4636) (33.3273, 68.3784) (33.4575, 68.3677) (33.5239, 68.3622) knots 0 0 0 0 0.018679 0.038112 0.038112 0.038112 0.038112
  spline S119 degree 3 poles (33.5239, 68.3622) (33.5903, 68.3677) (33.7205, 68.3784) (33.8193, 68.4636) (33.8677, 68.5054) knots 0 0 0 0 0.019433 0.038112 0.038112 0.038112 0.038112
  spline S120 degree 3 poles (33.8677, 68.5054) (33.9067, 68.5542) (33.987, 68.6546) (33.9965, 68.7831) (34.0014, 68.8492) knots 0 0 0 0 0.018276 0.037667 0.037667 0.037667 0.037667
  line L236 (34.0014, 68.8492) -> (34.0014, 72.8411)
  line L237 (30.2673, 68.4768) -> (31.2414, 69.193)
  line L238 (31.2414, 69.193) -> (31.2414, 68.1616)
  line L239 (31.2414, 68.1616) -> (30.2673, 67.4454)
  line L240 (30.2673, 67.4454) -> (29.2932, 67.4454)
  line L241 (29.2932, 67.4454) -> (29.2932, 74.245)
  line L242 (29.2932, 74.245) -> (30.2673, 74.245)
  line L243 (30.2673, 74.245) -> (30.2673, 68.4768)
  line L244 (26.4092, 71.3895) -> (26.4283, 71.3704)
  spline S121 degree 3 poles (26.4283, 71.3704) (26.4485, 71.3833) (26.496, 71.4133) (26.5501, 71.4285) (26.5811, 71.4373) knots 0 0 0 0 0.007166 0.016755 0.016755 0.016755 0.016755
  spline S122 degree 3 poles (26.5811, 71.4373) (26.6184, 71.4428) (26.7038, 71.4555) (26.7903, 71.4561) (26.8389, 71.4564) knots 0 0 0 0 0.011312 0.025884 0.025884 0.025884 0.025884
  spline S123 degree 3 poles (26.8389, 71.4564) (26.923, 71.4513) (27.0904, 71.4413) (27.2413, 71.3684) (27.3164, 71.3322) knots 0 0 0 0 0.025023 0.049762 0.049762 0.049762 0.049762
  spline S124 degree 3 poles (27.3164, 71.3322) (27.3851, 71.2889) (27.5188, 71.2046) (27.6139, 71.0785) (27.6602, 71.0171) knots 0 0 0 0 0.024118 0.046985 0.046985 0.046985 0.046985
  spline S125 degree 3 poles (27.6602, 71.0171) (27.6812, 70.985) (27.7228, 70.9216) (27.7512, 70.8513) (27.7653, 70.8165) knots 0 0 0 0 0.011465 0.022689 0.022689 0.022689 0.022689
  spline S126 degree 3 poles (27.7653, 70.8165) (27.7779, 70.7737) (27.8059, 70.6796) (27.8228, 70.5828) (27.8321, 70.53) knots 0 0 0 0 0.013381 0.029441 0.029441 0.029441 0.029441
  spline S127 degree 3 poles (27.8321, 70.53) (27.8382, 70.4656) (27.8517, 70.3226) (27.8575, 70.1791) (27.8608, 70.1003) knots 0 0 0 0 0.019411 0.043077 0.043077 0.043077 0.043077
  spline S128 degree 3 poles (27.8608, 70.1003) (27.8635, 70) (27.8697, 69.7772) (27.8701, 69.5543) (27.8703, 69.4318) knots 0 0 0 0 0.030091 0.066859 0.066859 0.066859 0.066859
  spline S129 degree 3 poles (27.8703, 69.4318) (27.8701, 69.3307) (27.8698, 69.1492) (27.8635, 68.9678) (27.8608, 68.8874) knots 0 0 0 0 0.030322 0.054447 0.054447 0.054447 0.054447
  spline S130 degree 3 poles (27.8608, 68.8874) (27.8576, 68.8205) (27.8518, 68.6992) (27.8382, 68.5786) (27.8321, 68.5245) knots 0 0 0 0 0.02009 0.036411 0.036411 0.036411 0.036411
  spline S131 degree 3 poles (27.8321, 68.5245) (27.8228, 68.4773) (27.8055, 68.39) (27.7779, 68.3055) (27.7653, 68.2667) knots 0 0 0 0 0.014424 0.026659 0.026659 0.026659 0.026659
  spline S132 degree 3 poles (27.7653, 68.2667) (27.7482, 68.2306) (27.7128, 68.156) (27.6718, 68.0842) (27.6507, 68.047) knots 0 0 0 0 0.011959 0.024783 0.024783 0.024783 0.024783
  spline S133 degree 3 poles (27.6507, 68.047) (27.5822, 67.9481) (27.4462, 67.7517) (27.2446, 67.6236) (27.1445, 67.56) knots 0 0 0 0 0.035683 0.070878 0.070878 0.070878 0.070878
  spline S134 degree 3 poles (27.1445, 67.56) (27.0316, 67.5098) (26.8006, 67.4072) (26.5479, 67.3946) (26.4187, 67.3881) knots 0 0 0 0 0.036718 0.075159 0.075159 0.075159 0.075159
  spline S135 degree 3 poles (26.4187, 67.3881) (26.29, 67.3948) (26.0391, 67.408) (25.8127, 67.5166) (25.7024, 67.5695) knots 0 0 0 0 0.038232 0.074542 0.074542 0.074542 0.074542
  spline S136 degree 3 poles (25.7024, 67.5695) (25.6025, 67.6324) (25.4025, 67.7584) (25.2651, 67.9508) (25.1963, 68.047) knots 0 0 0 0 0.035054 0.070179 0.070179 0.070179 0.070179
  spline S137 degree 3 poles (25.1963, 68.047) (25.1751, 68.0842) (25.1342, 68.156) (25.0988, 68.2306) (25.0817, 68.2667) knots 0 0 0 0 0.012824 0.024783 0.024783 0.024783 0.024783
  spline S138 degree 3 poles (25.0817, 68.2667) (25.0668, 68.3053) (25.0346, 68.3886) (25.0218, 68.4771) (25.0149, 68.5245) knots 0 0 0 0 0.012383 0.026712 0.026712 0.026712 0.026712
  spline S139 degree 3 poles (25.0149, 68.5245) (25.006, 68.5785) (24.9862, 68.6987) (24.9801, 68.8204) (24.9767, 68.8874) knots 0 0 0 0 0.01641 0.036516 0.036516 0.036516 0.036516
  spline S140 degree 3 poles (24.9767, 68.8874) (24.9739, 68.9678) (24.9676, 69.1492) (24.9673, 69.3307) (24.9671, 69.4318) knots 0 0 0 0 0.024124 0.054447 0.054447 0.054447 0.054447
  spline S141 degree 3 poles (24.9671, 69.4318) (24.9673, 69.5281) (24.9677, 69.7032) (24.9739, 69.8782) (24.9767, 69.957) knots 0 0 0 0 0.02889 0.052537 0.052537 0.052537 0.052537
  spline S142 degree 3 poles (24.9767, 69.957) (24.9803, 70.02) (24.9871, 70.1385) (25.006, 70.2556) (25.0149, 70.3104) knots 0 0 0 0 0.018916 0.035561 0.035561 0.035561 0.035561
  spline S143 degree 3 poles (25.0149, 70.3104) (25.0218, 70.3567) (25.0354, 70.4471) (25.0601, 70.535) (25.0722, 70.5778) knots 0 0 0 0 0.014052 0.027371 0.027371 0.027371 0.027371
  spline S144 degree 3 poles (25.0722, 70.5778) (25.0828, 70.6177) (25.1052, 70.7014) (25.1337, 70.7833) (25.1486, 70.8261) knots 0 0 0 0 0.012397 0.025986 0.025986 0.025986 0.025986
  line L245 (25.1486, 70.8261) -> (26.4283, 74.245)
  line L246 (26.4283, 74.245) -> (27.517, 74.245)
  line L247 (27.517, 74.245) -> (26.4092, 71.3895)
  spline S145 degree 3 poles (26.8962, 70.1098) (26.891, 70.1787) (26.8811, 70.3121) (26.7947, 70.4139) (26.753, 70.4632) knots 0 0 0 0 0.020137 0.039012 0.039012 0.039012 0.039012
  spline S146 degree 3 poles (26.753, 70.4632) (26.7034, 70.5022) (26.6051, 70.5796) (26.4805, 70.5911) (26.4187, 70.5969) knots 0 0 0 0 0.018476 0.036692 0.036692 0.036692 0.036692
  spline S147 degree 3 poles (26.4187, 70.5969) (26.3569, 70.5911) (26.2323, 70.5796) (26.134, 70.5022) (26.0845, 70.4632) knots 0 0 0 0 0.018216 0.036692 0.036692 0.036692 0.036692
  spline S148 degree 3 poles (26.0845, 70.4632) (26.0427, 70.4139) (25.9563, 70.3121) (25.9464, 70.1787) (25.9412, 70.1098) knots 0 0 0 0 0.018875 0.039012 0.039012 0.039012 0.039012
  line L248 (25.9412, 70.1098) -> (25.9412, 68.8492)
  spline S149 degree 3 poles (25.9412, 68.8492) (25.9464, 68.7804) (25.9563, 68.647) (26.0427, 68.5451) (26.0845, 68.4959) knots 0 0 0 0 0.020137 0.039012 0.039012 0.039012 0.039012
  spline S150 degree 3 poles (26.0845, 68.4959) (26.134, 68.4569) (26.2323, 68.3794) (26.3569, 68.3679) (26.4187, 68.3622) knots 0 0 0 0 0.018476 0.036692 0.036692 0.036692 0.036692
  spline S151 degree 3 poles (26.4187, 68.3622) (26.4805, 68.3679) (26.6051, 68.3794) (26.7034, 68.4569) (26.753, 68.4959) knots 0 0 0 0 0.018215 0.036692 0.036692 0.036692 0.036692
  spline S152 degree 3 poles (26.753, 68.4959) (26.7947, 68.5451) (26.8811, 68.647) (26.891, 68.7804) (26.8962, 68.8492) knots 0 0 0 0 0.018875 0.039012 0.039012 0.039012 0.039012
  line L249 (26.8962, 68.8492) -> (26.8962, 70.1098)
  dimension "d148" = 5
  dimension "d149" = 25
  dimension "d150" = 5
  dimension "d151" = 40
  constraint horizontal L99
  constraint vertical L100
  constraint horizontal L101
  constraint vertical L102
  constraint horizontal L103
  constraint vertical L104
  constraint horizontal L105
  constraint vertical L106
  constraint horizontal L107
  constraint vertical L108
  constraint horizontal L109
  constraint vertical L110
  constraint horizontal L111
  constraint vertical L112
  constraint horizontal L113
  constraint vertical L114
  constraint midpoint L105 L111.start
  constraint horizontal L115
  constraint vertical L116
  constraint horizontal L117
  constraint vertical L118
  constraint horizontal L119
  constraint vertical L120
  constraint horizontal L121
  constraint vertical L122
  constraint horizontal L123
  constraint vertical L124
  constraint horizontal L125
  constraint vertical L126
  constraint coincident L110 L124.end
  constraint horizontal L127
  constraint vertical L128
  constraint horizontal L129
  constraint vertical L130
  constraint horizontal L131
  constraint vertical L132
  constraint horizontal L133
  constraint vertical L134
  constraint horizontal L135
  constraint vertical L136
  constraint horizontal L137
  constraint vertical L138
  measures "d148" distance of L99.start L99.end
  measures "d149" distance of L99.start L101.end
  measures "d150" distance of L101.end L105.end
  measures "d151" distance of L101.end L103.end
extrude "Extrude17" cut sketch "Sketch13" against normal blind 1.5 contours L99 L132 L133 L134 L135 L136 L137 L138 L139 L140 L141 L142 L143 L144 L145 L152 | L99 L100 L126 L128 L129 L130 L131 L148 L151 | L104 L116 L117 L118 L119 L120 L121 L122 L123 L124 L125 L127 L146 L150 | L105 L106 L107 L108 L109 L110 L111 L112 L113 L114 L115 L116 L149 bodies 1
mirror "Mirror1" about plane through (0, 0, 0) normal (1, 0, 0) of bodies 1 makes body 2
hidden bodies 1
equation "d31 = d30 + 4 mm"
equation "d37 = d30"
equation "d38 = d31"
equation "d45 = d44 + 4 mm"
equation "d46 = d44"
equation "d47 = d45"
equation "d54 = d53 + 4 mm"
equation "d59 = d53"
equation "d60 = d54"
equation "d66 = d65 + 4 mm"
equation "d67 = d65"
equation "d68 = d66"
equation "d76 = d75 + 4 mm"
equation "d77 = d75"
equation "d78 = d76"
equation "d85 = d84 + 4 mm"
equation "d87 = d84"
equation "d88 = d85"
equation "d92 = 183.540758 mm / 2"
equation "d94 = d84"
equation "d95 = d85"
equation "d103 = 4.1 mm + 4 mm"
equation "d104 = d102"
equation "d105 = d103"
equation "d110 = d25 - 0.3 mm"
equation "d111 = d109 + 1 mm"
equation "d112 = d110 - 1 mm"
equation "d120 = d119 + 4 mm"
equation "d130 = d129 + 4 mm"
